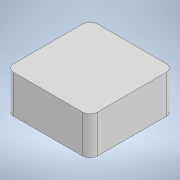
# Autodesk Inventor part: box
Saved by Autodesk Inventor 2022 (Build 260153000, 153)
## iProperties
Created: 2021-07-02
Part Number: box
Material: Generic
Document SubType Name: Modeling
Designer: 91810
Density: 1 g/cm^3
Appearance: Default
Author: 91810
Autodesk Inventor part; units mm, degrees
ref_plane "YZ Plane" through (0, 0, 0) normal (1, 0, 0) x (0, 1, 0)
ref_plane "XZ Plane" through (0, 0, 0) normal (0, 1, 0) x (-1, 0, 0)
ref_plane "XY Plane" through (0, 0, 0) normal (0, 0, 1) x (1, 0, 0)
sketch "Sketch1" plane through (0, 0, 0) normal (0, 1, 0) x (-1, 0, 0)
  line L0 (7.4919, 7.8851) -> (-12.5081, 7.8851)
  line L1 (-12.5081, 7.8851) -> (-12.5081, -12.1149)
  line L2 (-12.5081, -12.1149) -> (7.4919, -12.1149)
  line L3 (7.4919, -12.1149) -> (7.4919, 7.8851)
  line L4 (8.4919, 8.8851) -> (-13.5081, 8.8851)
  line L5 (-13.5081, 8.8851) -> (-13.5081, -13.1149)
  line L6 (-13.5081, -13.1149) -> (8.4919, -13.1149)
  line L7 (8.4919, -13.1149) -> (8.4919, 8.8851)
  point P0 (0, 0)
  dimension "d0" = 20
  dimension "d1" = 20
  dimension "d2" = 22
  dimension "d3" = 22
  dimension "d4" = 1
  dimension "d5" = 1
  constraints: 16 end point, 4 parallel, 2 horizontal, 2 perpendicular
  measures "d0" distance of L2.end L1.end
  measures "d1" distance of L1.end L0.end
  measures "d2" distance of L6.end L5.end
  measures "d3" distance of L5.end L4.end
  measures "d4" distance between parallel lines of L0 L4
  measures "d5" distance between parallel lines of L3 L7
extrude "Extrusion1" add sketch "Sketch1" along normal blind 10 contours L3 L2 L1 L0 | L7 L6 L5 L4
sketch "Sketch2" plane through (0, 0, 0) normal (0, 1, 0) x (-1, 0, 0)
  line L0 (7.4919, 7.8851) -> (-12.5081, 7.8851)
  line L1 (-12.5081, 7.8851) -> (-12.5081, -12.1149)
  line L2 (-12.5081, -12.1149) -> (7.4919, -12.1149)
  line L3 (7.4919, -12.1149) -> (7.4919, 7.8851)
  line L4 (8.4919, -13.1149) -> (8.4919, 8.8851) projected
  line L5 (8.4919, 8.8851) -> (-13.5081, 8.8851) projected
  point P0 (0, 0)
  dimension "d8" = 20
  dimension "d9" = 20
  dimension "d10" = 1
  dimension "d11" = 1
  constraints: 8 end point, 2 parallel, 1 horizontal, 1 perpendicular
  measures "d8" distance of L2.end L1.end
  measures "d9" distance of L1.end L0.end
  measures "d10" distance between parallel lines of L4 L3
  measures "d11" distance between parallel lines of L5 L0
extrude "Extrusion2" cut sketch "Sketch2" along normal blind 9
fillet "Fillet1" radius 2 4 edges at (-8.4919, 5, 8.8851) (-8.4919, 5, -13.1149) (13.5081, 5, -13.1149) (13.5081, 5, 8.8851)
body "Solid1"
